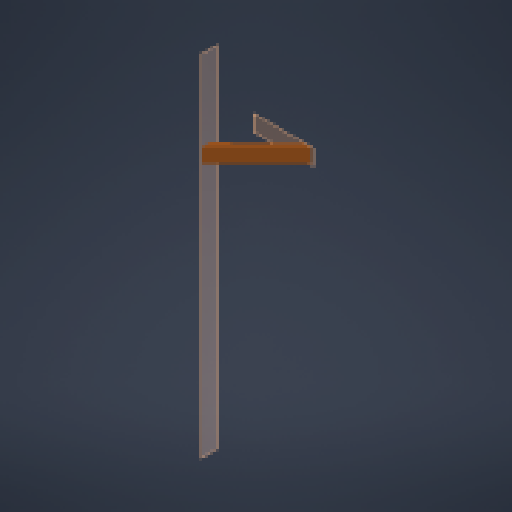
# Autodesk Inventor part: Top Diagonals
Saved by Autodesk Inventor 2027 (Build 310192000, 192)
## iProperties
Created: 2026-08-07
Part Number: Top Diagonals
Material: Generic
Document SubType Name: Modeling
Designer: lucas
Density: 1 g/cm^3
Appearance: Default
Author: lucas
Autodesk Inventor part; units mm, degrees
ref_plane "YZ Plane" through (0, 0, 0) normal (1, 0, 0) x (0, 1, 0)
ref_plane "XZ Plane" through (0, 0, 0) normal (0, 1, 0) x (-1, 0, 0)
ref_plane "XY Plane" through (0, 0, 0) normal (0, 0, 1) x (1, 0, 0)
ref_plane "Work Plane1" through (0, 0, 0) normal (0, 0, 1) x (1, 0, 0)
sketch "Sketch1" plane through (0, 0, 0) normal (0, 0, 1) x (1, 0, 0)
  line L0 (190.5, -50.8) -> (190.5, 50.8) projected
  line L1 (190.5, 50.8) -> (67.5314, 50.8) projected
  line L2 (190.5, 50.8) -> (139.7, 50.8)
  line L3 (139.7, 50.8) -> (139.7, -50.8)
  line L4 (139.7, -50.8) -> (190.5, -50.8)
  line L5 (190.5, -50.8) -> (190.5, 50.8)
  point P0 (0, 0)
  dimension "d0" = 50.8
  constraints: 8 end point, 2 parallel, 1 horizontal, 1 perpendicular
  measures "d0" distance of L3.end L4.end
ref_plane "Work Plane2" through (-190.5, -609.6, 330.2) normal (1, 0, 0) x (0, -1, 0)
sketch "Sketch2" plane through (-190.5, -609.6, 330.2) normal (1, 0, 0) x (0, -1, 0)
  line L0 (-1117.6, 50.8) -> (1117.6, 50.8) projected
  line L1 (1117.6, -50.8) -> (-1117.6, -50.8) projected
  line L2 (-558.8, 330.2) -> (-660.4, 330.2) projected
  line L3 (-662.9873, -50.8) -> (-558.8, -50.8)
  line L4 (-558.8, -50.8) -> (-558.8, 0)
  line L5 (-558.8, 0) -> (-662.9873, 0)
  line L6 (-662.9873, 0) -> (-662.9873, -50.8)
  point P0 (-609.6, 330.2)
  dimension "d1" = 50.8
  constraints: 8 end point, 2 parallel, 1 horizontal, 1 perpendicular, 1 point on line
  measures "d1" distance of L3.end L4.end
loft "Loft1" add profiles "Sketch1", "Sketch2"
body "Solid1"
